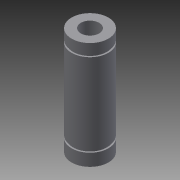
# Autodesk Inventor part: LinearBearing
Saved by Autodesk Inventor 2015 (Build 190159000, 159)
## iProperties
Created: 2017-01-04
Part Number: LinearBearing
Material: Generic
Document SubType Name: Modeling
Designer: Ernest
Density: 1 g/cm^3
Appearance: Default
Mass: 2.94352 g
Surface Area: 22.1671 cm^2
Volume: 2.94352 cm^3
Author: Ernest
Autodesk Inventor part; units mm, degrees
ref_plane "YZ Plane" through (0, 0, 0) normal (1, 0, 0) x (0, 1, 0)
sketch "Sketch1" plane through (0, 0, 0) normal (0, 0, 1) x (1, 0, 0)
  circle A0 centre (0, 0) radius 3
  circle A1 centre (0, 0) radius 6
  dimension "d0" = 6
  dimension "d1" = 12
  constraints: 2 centre point, 2 coincident
  measures "d0" diameter of A0
  measures "d1" diameter of A1
extrude "Extrusion1" add sketch "Sketch1" along normal blind 35
ref_plane "Work Plane1" through (0, 0, 31) normal (0, 0, 1) x (1, 0, 0)
ref_plane "Work Plane2" through (0, 0, 4) normal (0, 0, -1) x (-1, 0, 0)
sketch "Sketch2" plane through (0, 0, 31) normal (0, 0, 1) x (1, 0, 0)
  circle A0 centre (0, 0) radius 3 projected
  circle A1 centre (0, 0) radius 6 projected
  circle A2 centre (0, 0) radius 5.5
  circle A3 centre (0, 0) radius 6
  dimension "d6" = 11
  constraints: 2 centre point, 2 coincident
  measures "d6" diameter of A2
extrude "Extrusion2" cut sketch "Sketch2" along normal blind 0.7 contours A1
sketch "Sketch3" plane through (0, 0, 4) normal (0, 0, -1) x (-1, 0, 0)
  circle A0 centre (0, 0) radius 3 projected
  circle A1 centre (0, 0) radius 6 projected
  circle A2 centre (0, 0) radius 5.5
  circle A3 centre (0, 0) radius 6
  dimension "d9" = 11
  constraints: 2 centre point, 2 coincident
  measures "d9" diameter of A2
extrude "Extrusion3" cut sketch "Sketch3" against normal blind 0.7 contours A1
body "Solid1"
